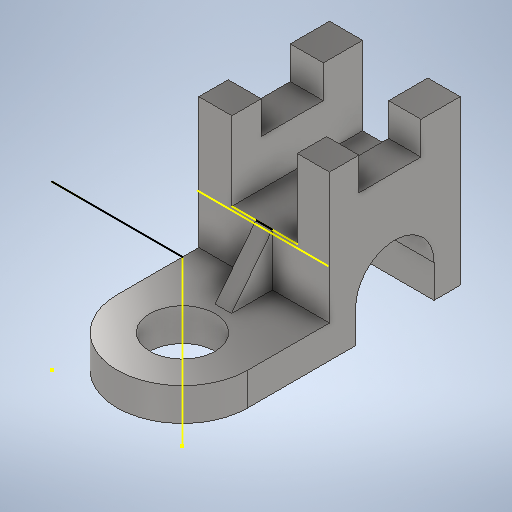
# Autodesk Inventor part: Baitap1
Saved by Autodesk Inventor 2025.2 (Build 292293000, 293)
## iProperties
Created: 2024-12-04
Part Number: Baitap1
Material: Steel, Carbon
Document SubType Name: Modeling
Designer: hongquan
Density: 7.85 g/cm^3
Appearance: Semi-Polished
Mass: 3265.21 g
Surface Area: 654.382 cm^2
Volume: 415.95 cm^3
Author: hongquan
Autodesk Inventor part; units mm, degrees
ref_plane "YZ Plane" through (0, 0, 0) normal (1, 0, 0) x (0, 1, 0)
ref_plane "XZ Plane" through (0, 0, 0) normal (0, 1, 0) x (-1, 0, 0)
ref_plane "XY Plane" through (0, 0, 0) normal (0, 0, 1) x (1, 0, 0)
sketch "Sketch1" plane through (0, 0, 0) normal (1, 0, 0) x (0, 1, 0)
  line L0 (0, 0) -> (100, 0)
  line L1 (100, 0) -> (100, -170)
  line L2 (100, -170) -> (0, -170)
  line L3 (0, -170) -> (0, 0)
  dimension "d0" = 100
  dimension "d1" = 170
  constraints: 8 end point, 2 parallel, 1 horizontal, 1 perpendicular
  measures "d0" distance of L1.end L2.end
  measures "d1" distance of L2.end L0.start
extrude "Extrusion1" add sketch "Sketch1" along normal blind 80
sketch "Sketch2" plane through (80, 0, 0) normal (1, 0, 0) x (0, 0, -1)
  line L0 (0, 0) -> (40, 0)
  line L1 (0, 0) -> (170, 0) construction
  line L2 (40, 0) -> (170, 0) construction
  line L3 (170, 0) -> (130, 0)
  line L4 (0, 100) -> (0, 0) projected
  line L5 (0, 0) -> (0, 20) construction
  line L6 (130, 0) -> (130, 20)
  arc A0 (154, 20) -> (106, 20) centre (130, 20) ccw
  line L7 (106, 20) -> (106, 0)
  line L8 (154, 20) -> (154, 0)
  line L9 (106, 0) -> (154, 0)
  dimension "d4" = 40
  dimension "d5" = 40
  dimension "d6" = 20
  dimension "d7" = 48
  dimension "d8" = 20
  constraints: 16 end point, 5 point on line, 2 coincident, 2 collinear, 2 perpendicular, 2 point on circle, 2 tangent, 1 centre point, 1 vertical
  measures "d4" distance of L0.start L0.end
  measures "d5" distance of L1.end L3.end
  measures "d6" distance of L0.start L5.end
  measures "d7" diameter of A0
  measures "d8" distance of L8.start L8.end
sketch "Sketch3" plane through (80, 0, 0) normal (1, 0, 0) x (0, 0, -1)
  line L0 (170, 100) -> (0, 100) projected
  line L1 (170, 100) -> (170, 80) construction
  line L2 (170, 0) -> (170, 100) construction
  line L3 (170, 100) -> (146, 100)
  line L4 (146, 100) -> (108, 100)
  line L5 (108, 100) -> (90, 100)
  line L6 (170, 100) -> (170, 80)
  line L7 (170, 0) -> (170, 100) construction
  line L8 (0, 100) -> (0, 0) projected
  line L9 (0, 19.805) -> (170, 19.805) construction
  line L10 (90, 100) -> (90, 19.805)
  line L11 (0, 19.805) -> (90, 19.805)
  line L12 (108, 100) -> (108, 80)
  line L13 (108, 80) -> (146, 80)
  line L14 (146, 80) -> (146, 100)
  line L15 (90, 100) -> (90, 52) construction
  line L16 (90, 19.805) -> (65, 19.805) construction
  line L17 (90, 52) -> (65, 19.805)
  dimension "d9" = 20
  dimension "d10" = 24
  dimension "d11" = 38
  dimension "d12" = 18
  dimension "d22" = 48
  dimension "d23" = 25
  constraints: 28 end point, 9 point on line, 4 perpendicular, 2 collinear, 2 horizontal, 1 vertical
  measures "d9" distance of L0.start L1.end
  measures "d10" distance of L0.start L3.end
  measures "d11" distance of L3.end L4.end
  measures "d12" distance of L4.end L5.end
  measures "d22" distance of L5.end L15.end
  measures "d23" distance of L10.end L16.end
extrude "Extrusion2" cut sketch "Sketch2" against normal blind 80
extrude "Extrusion3" cut sketch "Sketch3" against normal blind 80 contours L14 L13 L12 L0
sketch "Sketch4" plane through (0, 0, 0) normal (0, 0, 1) x (1, 0, 0)
  line L0 (80, 100) -> (0, 100) projected
  line L1 (0, 100) -> (0, 52)
  line L2 (0, 0) -> (0, 100) projected
  line L3 (0, 52) -> (80.2195, 52)
  line L4 (80.2195, 52) -> (80.2195, 100)
  line L5 (80.2195, 100) -> (60.2195, 100)
  line L6 (60.2195, 100) -> (20.2195, 100)
  line L7 (20.2195, 100) -> (0, 100)
  line L8 (20.2195, 100) -> (20.2195, 52)
  line L9 (60.2195, 100) -> (60.2195, 52)
  dimension "d17" = 48
  dimension "d18" = 20
  dimension "d19" = 40
  constraints: 16 end point, 5 perpendicular, 4 point on line, 1 collinear, 1 vertical
  measures "d17" distance of L0.end L1.end
  measures "d18" distance of L4.end L5.end
  measures "d19" distance of L5.end L6.end
extrude "Extrusion4" cut sketch "Sketch4" against normal blind 170 contours L9 L3 L8 L0
sketch "Sketch5" plane through (80, 0, 0) normal (1, 0, 0) x (0, 0, -1)
  point P0 (0, 0)
sketch "Sketch6" plane through (0, 0, 0) normal (0, 0, 1) x (1, 0, 0)
  line L0 (0, 100) -> (20.2195, 100) projected
  line L1 (80, 100) -> (80, 0) projected
  line L2 (0, 100) -> (80, 100)
  point P0 (0, 0)
  constraints: 2 end point, 1 horizontal
ref_plane "Work Plane1" through (40, 0, 0) normal (-1, 0, 0) x (0, 0, 1)
sketch "Sketch7" plane through (40, 0, 0) normal (-1, 0, 0) x (0, 0, 1)
  line L0 (-170, 0) -> (-170, 100) projected
  line L1 (-170, 100) -> (-90, 100)
  line L2 (-108, 100) -> (0, 100) projected
  line L3 (-90, 100) -> (-90, 52)
  line L4 (-90, 52) -> (-90, 0)
  line L5 (0, 0) -> (0, 20)
  line L6 (0, 100) -> (0, 0) projected
  line L7 (0, 20) -> (-90, 20)
  line L8 (-90, 20) -> (-65, 20)
  line L9 (-65, 20) -> (-90, 52)
  dimension "d24" = 80
  dimension "d25" = 48
  dimension "d26" = 20
  dimension "d27" = 25
  constraints: 14 end point, 5 point on line, 2 perpendicular
  measures "d24" distance of L0.end L1.end
  measures "d25" distance of L1.end L3.end
  measures "d26" distance of L5.start L5.end
  measures "d27" distance of L7.end L8.end
extrude "Extrusion5" cut sketch "Sketch7" along normal mid plane 100
extrude "Extrusion6" add sketch "Sketch7" along normal mid plane 10 contours L9 L7 L4
sketch "Sketch9" plane through (0, 100, -90) normal (0, 0, 1) x (1, 0, 0)
  line L0 (20.2195, -48) -> (60.2195, -48) projected
  line L1 (37.4638, -48) -> (42.5225, -48)
  point P0 (0, -100)
  constraints: 2 end point, 2 point on line
sketch "Sketch10" plane through (0, 20, 0) normal (0, 1, 0) x (1, 0, 0)
  line L0 (0, 0) -> (80, 0) projected
  line L1 (40, 0) -> (40, 40) construction
  circle A0 centre (40, 40) radius 20
  arc A1 (40, 0) -> (80, 40) centre (40, 40) ccw
  line L2 (0, 0) -> (0, 106) projected
  arc A2 (0, 40) -> (40, 0) centre (40, 40) ccw
  line L3 (0, 40) -> (0, 0)
  line L4 (40, 0) -> (0, 0)
  line L5 (80, 0) -> (80, 106) projected
  line L6 (40, 0) -> (80, 0)
  line L7 (80, 0) -> (80, 40)
  dimension "d32" = 40
  dimension "d33" = 40
  constraints: 10 end point, 5 point on circle, 3 centre point, 3 coincident, 2 tangent, 2 vertical, 1 horizontal, 1 midpoint, 1 perpendicular, 1 point on line
  measures "d32" distance of L1.start L1.end
  measures "d33" diameter of A0
extrude "Extrusion7" cut sketch "Sketch10" against normal blind 20
sketch "Sketch11" plane through (35, 52, -90) normal (0, 0.615644, 0.7880244) x (1, 0, 0)
  line L0 (0, 0) -> (10, 0) projected
  line L1 (0, 0) -> (10, 0)
  line L2 (10, 0) -> (0, 0)
  line L3 (45, -1.576) -> (-35, -1.576) projected
  point P0 (-35, -96.3852)
  constraints: 4 end point, 1 horizontal, 1 parallel
body "Solid1"
